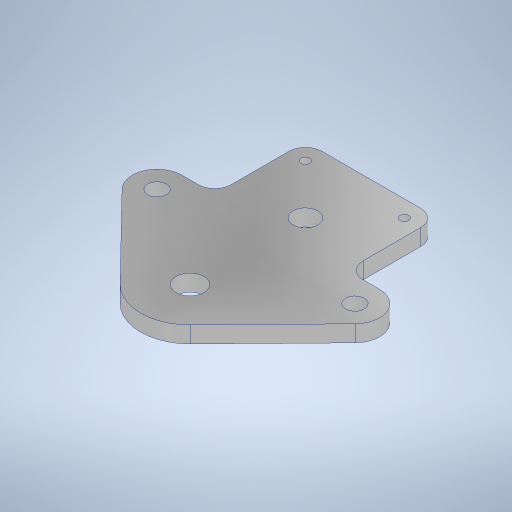
# Autodesk Inventor part: Upright (Top)
Saved by Autodesk Inventor 2023.1 (Build 271208000, 208)
## iProperties
Created: 2022-11-17
Part Number: Upright (Top)
Material: Aluminum 6061
Document SubType Name: Modeling
Designer: Nathan Cai
Density: 2.7 g/cm^3
Appearance: Aluminum - Flat
Author: Nathan Cai
Autodesk Inventor part; units mm, degrees
ref_plane "YZ Plane" through (0, 0, 0) normal (1, 0, 0) x (0, 1, 0)
ref_plane "XZ Plane" through (0, 0, 0) normal (0, 1, 0) x (-1, 0, 0)
ref_plane "XY Plane" through (0, 0, 0) normal (0, 0, 1) x (1, 0, 0)
sketch "Sketch1" plane through (0, 0, 0) normal (0, 1, 0) x (-1, 0, 0)
  circle A0 centre (0, 0) radius 38.1 construction
  line L0 (-38.1, 0) -> (38.1, 0) construction
  circle A1 centre (-38.1, 0) radius 3.6195
  circle A2 centre (38.1, 0) radius 3.6195
  line L1 (0, 0) -> (0, -38.1) construction
  circle A3 centre (0, -19.05) radius 22.225 construction
  circle A4 centre (0, -19.05) radius 4.7625
  line L2 (0, 0) -> (0, 38.1) construction
  circle A5 centre (0, 25.4) radius 5.3975
  circle A6 centre (0, 25.4) radius 19.05
  circle A7 centre (-38.1, 0) radius 9.525
  circle A8 centre (38.1, 0) radius 9.525
  circle A9 centre (-19.05, -38.1) radius 1.7526
  circle A10 centre (19.05, -38.1) radius 1.7526
  circle A11 centre (-19.05, -38.1) radius 6.35
  circle A12 centre (19.05, -38.1) radius 6.35
  line L3 (-44.9165, 6.6529) -> (-13.633, 38.7058)
  line L4 (-25.4, -38.1) -> (-25.4, 0)
  line L5 (-38.1, -9.525) -> (-25.4, -9.525)
  line L6 (44.9165, 6.6529) -> (13.633, 38.7058)
  line L7 (25.4, -38.1) -> (25.4, 0)
  line L8 (38.1, -9.525) -> (25.4, -9.525)
  line L9 (-19.05, -44.45) -> (19.05, -44.45)
  point P0 (25.4, -38.1)
  dimension "d11" = 38.1
  dimension "d18" = 12.7
  dimension "d0" = 76.2
  dimension "d1" = 7.239
  dimension "d2" = 7.239
  dimension "d3" = 44.45
  dimension "d4" = 9.525
  dimension "d5" = 19.05
  dimension "d9" = 10.795
  dimension "d10" = 44.45
  dimension "d12" = 19.05
  dimension "d13" = 19.05
  dimension "d14" = 3.5052
  dimension "d15" = 38.1
  dimension "d16" = 19.05
  dimension "d17" = 12.7
  constraints: 20 end point, 11 centre point, 9 coincident, 8 point on circle, 7 symmetric about line, 4 point on line, 4 tangent, 3 midpoint, 2 horizontal, 2 perpendicular, 2 vertical, 8 other
  measures "d0" diameter of A0
  measures "d1" diameter of A1
  measures "d2" diameter of A2
  measures "d3" diameter of A3
  measures "d4" diameter of A4
  measures "d5" distance from line of L0 A3.centre
  measures "d9" diameter of A5
  measures "d10" distance of A3.centre A5.centre
  measures "d12" diameter of A7
  measures "d13" diameter of A8
  measures "d14" diameter of A9
  measures "d15" vertical distance of point (0, 0) A9.centre
  measures "d16" horizontal distance of point (0, 0) A9.centre
  measures "d17" diameter of A11
extrude "Extrusion1" add sketch "Sketch1" along normal blind 6.35
fillet "Fillet1" radius 6.35 2 edges at (25.4, 3.175, -9.525) (-25.4, 3.175, -9.525)
equation "\"d2\" = d1"
body "Solid1"
